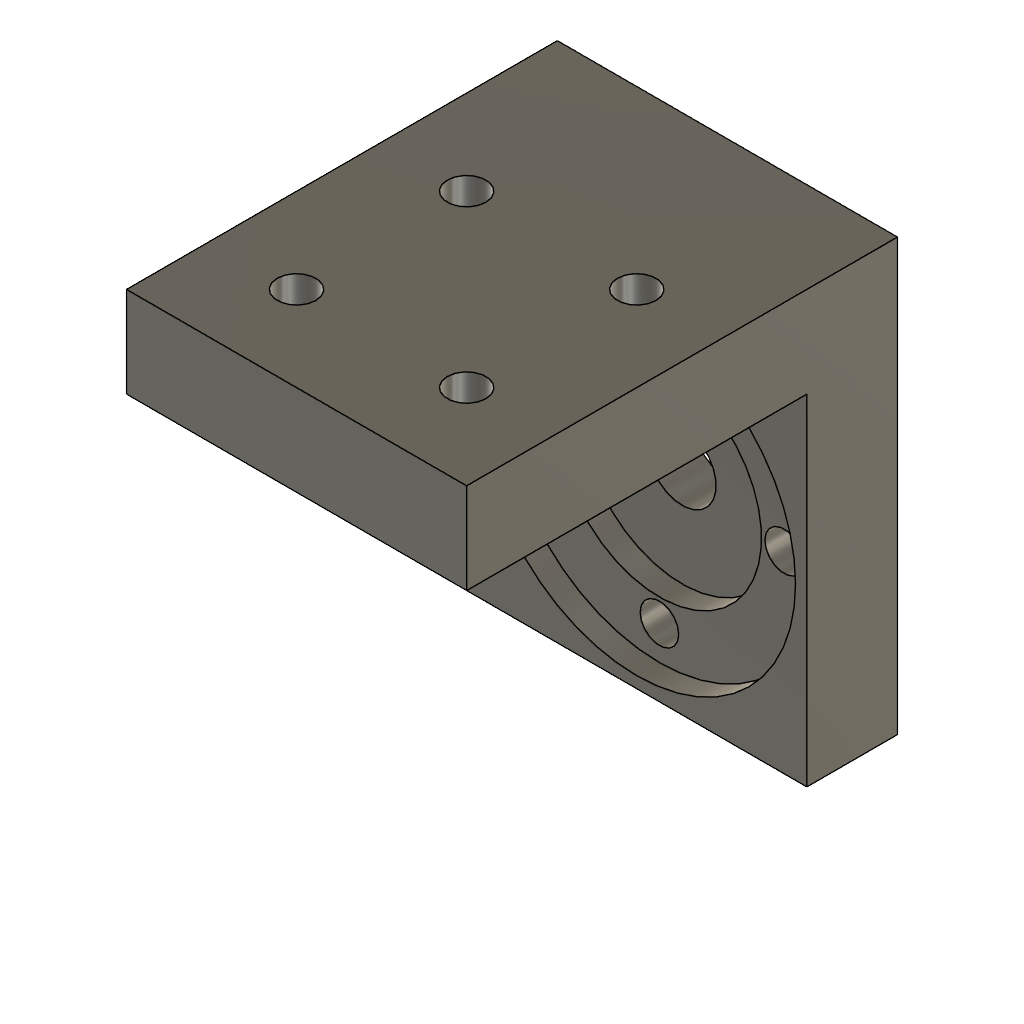
A4 (Autodesk Fusion 360 design; units mm, degrees)
part number: 2026-09-15-11-31-06-192
Autodesk Fusion 360 part; units mm, degrees
sketch "Sketch1" plane through (0, 0, 0) normal (0, 1, 0) x (1, 0, 0)
  line L0 (0, 0) -> (0, -30)
  line L1 (0, -30) -> (30, -30)
  line L2 (30, -30) -> (30, 0)
  line L3 (30, 0) -> (0, 0)
  dimension "d1" = 30
  dimension "d2" = 30
  constraint coincident L0.start L3.end
  constraint vertical L0
  constraint perpendicular L0 L1
  constraint perpendicular L1 L2
  constraint perpendicular L0 L3
  measures "d1" distance of L0.start L0.end
  measures "d2" distance of L0.end L1.end
extrude "Extrude1" add sketch "Sketch1" along normal blind 8
sketch "Sketch2" plane through (0, 0, 0) normal (0, -1, 0) x (1, 0, 0)
  line L0 (0, 0) -> (30, 0)
  line L1 (30, 0) -> (30, 30)
  line L2 (30, 30) -> (0, 30)
  line L3 (0, 30) -> (0, 0)
  circle A0 centre (15, 15) radius 14
  dimension "d5" = 28
  measures "d5" diameter of A0
extrude "Extrude2" cut sketch "Sketch2" along normal blind 2 and the other way blind 2 contours A0
sketch "Sketch4" plane through (0, 2, 0) normal (0, -1, 0) x (1, 0, 0)
  circle A0 centre (15, 15) radius 3
  dimension "d10" = 6
  measures "d10" diameter of A0
extrude "Extrude3" cut sketch "Sketch4" against normal blind 6
sketch "Sketch7" plane through (0, 0, 0) normal (1, 0, 0) x (0, 1, 0)
  line L0 (8, 30) -> (8, 38)
  line L1 (8, 38) -> (-30, 38)
  line L2 (8, 30) -> (-30, 30)
  line L3 (-30, 30) -> (-30, 38)
  dimension "d40" = 8
  dimension "d41" = 38
  constraint vertical L0
  constraint perpendicular L0 L1
  constraint perpendicular L0 L2
  measures "d40" distance of L0.start L0.end
  measures "d41" distance of L0.end L1.end
sketch "Sketch8" plane through (0, 2, 0) normal (0, -1, 0) x (1, 0, 0)
  circle A0 centre (15, 15) radius 3
  circle A1 centre (15, 15) radius 14
sketch "Sketch10" plane through (0, 2, 0) normal (0, -1, 0) x (1, 0, 0)
  circle A0 centre (15, 4) radius 1.7
  circle A1 centre (15, 26) radius 1.7
  circle A2 centre (4, 15) radius 1.7
  circle A3 centre (26, 15) radius 1.7
  dimension "d31" = 3.4
  dimension "d32" = 3.4
  dimension "d33" = 3.4
  dimension "d34" = 3.4
  measures "d31" diameter of A0
  measures "d32" diameter of A1
  measures "d33" diameter of A2
  measures "d34" diameter of A3
extrude "Extrude5" cut sketch "Sketch10" against normal blind 6
sketch "Sketch11" plane through (0, 2, 0) normal (0, -1, 0) x (1, 0, 0)
  circle A0 centre (15, 15) radius 9
  dimension "d37" = 18
  measures "d37" diameter of A0
extrude "Extrude6" cut sketch "Sketch11" against normal blind 2
extrude "Extrude7" add sketch "Sketch7" along normal blind 30
sketch "Sketch14" plane through (0, 0, 30) normal (0, 0, -1) x (1, 0, 0)
  line L0 (0, 0) -> (30, 0)
  line L1 (30, 0) -> (30, 30)
  line L2 (30, 30) -> (0, 30)
  line L3 (0, 30) -> (0, 0)
  circle A0 centre (7.5, 7.5) radius 1.7
  circle A1 centre (22.5, 7.5) radius 1.7
  circle A2 centre (7.5, 22.5) radius 1.7
  circle A3 centre (22.5, 22.5) radius 1.7
  dimension "d46" = 3.4
  dimension "d47" = 3.4
  dimension "d48" = 3.4
  dimension "d49" = 3.4
  measures "d46" diameter of A0
  measures "d47" diameter of A1
  measures "d48" diameter of A2
  measures "d49" diameter of A3
extrude "Extrude8" cut sketch "Sketch14" against normal blind 8 contours A0 | A1 | A2 | A3
equation "d1 = feature1Height"
equation "d2 = mountWidth"
equation "d5 = motorDC"
equation "d10 = shaftDiameter"
equation "d31 = boltClearance"
equation "d32 = boltClearance"
equation "d33 = boltClearance"
equation "d34 = boltClearance"
equation "d40 = plateThickness"
equation "d41 = feature2Length"
equation "d46 = boltClearance"
equation "d47 = boltClearance"
equation "d48 = boltClearance"
equation "d49 = boltClearance"
equation "mountWidth = 30 mm"
equation "feature1Height = 30 mm"
equation "feature2Length = 38 mm"
equation "plateThickness = 8 mm"
equation "motorBCD = 22 mm"
equation "boltClearance = 3.4 mm"
equation "shaftDiameter = 6 mm"
equation "pilotDiameter = 18 mm"
equation "pilotDepth = 2 mm"
equation "wallHoleOffset = 7.5 mm"
equation "motorDC = 28 mm"
